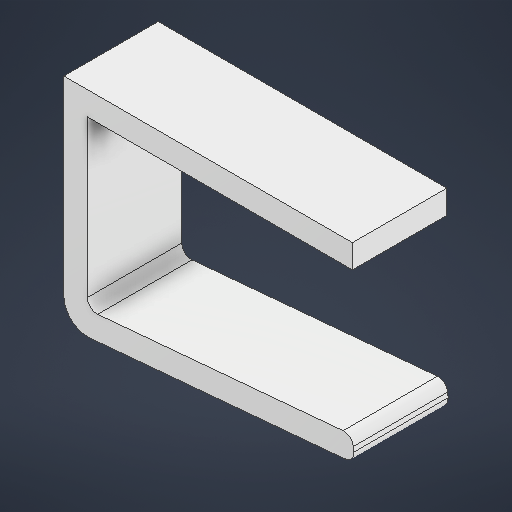
# Autodesk Inventor part: mpalanteza_clips
Saved by Autodesk Inventor 2026.1 (Build 301233020, 233B)
## iProperties
Created: 2026-02-17
Part Number: mpalanteza_clips
Material: ABS Plastic
Document SubType Name: Modeling
Designer: ar_mi
Density: 1.06 g/cm^3
Appearance: Smooth - White
Author: ar_mi
## iProperties of the stored document mpalanteza_clips_3DPrint.ipt
Created: 2026-02-18
Part Number: mpalanteza_clips_3DPrint
Material: Generic
Document SubType Name: Modeling
Designer: ar_mi
Density: 1 g/cm^3
Appearance: Default
Author: ar_mi
Autodesk Inventor part; units mm, degrees
ref_plane "YZ Plane" through (0, 0, 0) normal (1, 0, 0) x (0, 1, 0)
ref_plane "XZ Plane" through (0, 0, 0) normal (0, 1, 0) x (-1, 0, 0)
ref_plane "XY Plane" through (0, 0, 0) normal (0, 0, 1) x (1, 0, 0)
sketch "Sketch1" plane through (0, 0, 0) normal (0, 0, 1) x (1, 0, 0)
  line L0 (0, 0) -> (-56, 0)
  line L1 (-56, 0) -> (-56, -35)
  line L2 (-56, -35) -> (-56, -32)
  line L3 (-56, -35) -> (0, -30)
  dimension "d0" = 56
  dimension "d1" = 35
  dimension "d3" = 30
  constraints: 8 end point, 1 horizontal, 1 point on line, 1 vertical
  measures "d0" distance of L0.start L0.end
  measures "d1" distance of L0.end L1.end
  measures "d3" distance of L3.end L0.start
sketch "Sketch2" plane through (0, 0, 0) normal (1, 0, 0) x (0, 1, 0)
  line L0 (5.1629, 10) -> (0.1629, 10)
  line L1 (0.1629, 10) -> (0.1629, -10)
  line L2 (0.1629, -10) -> (5.1629, -10)
  line L3 (5.1629, -10) -> (5.1629, 10)
  line L4 (5.1629, 10) -> (0.1629, -10) construction
  line L5 (0.1629, 10) -> (5.1629, -10) construction
  point P0 (0, 0)
  point P1 (2.6629, 0)
  dimension "d4" = 5
  dimension "d5" = 20
  constraints: 12 end point, 2 midpoint, 2 parallel, 1 horizontal, 1 perpendicular
  measures "d4" distance of L2.end L1.end
  measures "d5" distance of L0.end L1.end
sweep "Sweep1" add profiles "Sketch2" path "Sketch1" path curves L0 L1 L3
fillet "Fillet1" radius 5 1 edges at (-61.1629, -40.6444, 0)
fillet "Fillet2" radius 2 1 edges at (-56.1629, -35.178, 0)
fillet "Fillet3" radius 2 2 edges at (0.0145, -30.1622, 0) (0.4591, -35.1424, 0)
body "Solid1"
